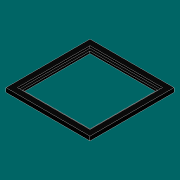
# Autodesk Inventor part: mirrorBackFrame
Saved by Autodesk Inventor 2016 (Build 200138000, 138)
## iProperties
Created: 2015-12-22
Part Number: mirrorBackFrame
Material: ABS Plastic
Document SubType Name: Modeling
Designer: sawai
Density: 1.06 g/cm^3
Appearance: Smooth - Black
Author: sawai
Autodesk Inventor part; units mm, degrees
ref_plane "YZ Plane" through (0, 0, 0) normal (1, 0, 0) x (0, 1, 0)
ref_plane "XZ Plane" through (0, 0, 0) normal (0, 1, 0) x (-1, 0, 0)
ref_plane "XY Plane" through (0, 0, 0) normal (0, 0, 1) x (1, 0, 0)
sketch "Sketch1" plane through (0, 0, 0) normal (0, 0, 1) x (1, 0, 0)
  line L0 (-57.15, 57.15) -> (57.15, 57.15) projected
  line L1 (57.15, 57.15) -> (57.15, -57.15) projected
  line L2 (57.15, -57.15) -> (-57.15, -57.15) projected
  line L3 (-57.15, -57.15) -> (-57.15, 57.15) projected
  line L4 (-63.5, -63.5) -> (63.5, -63.5) projected
  line L5 (63.5, -63.5) -> (63.5, 63.5) projected
  line L6 (63.5, 63.5) -> (-63.5, 63.5) projected
  line L7 (-63.5, 63.5) -> (-63.5, -63.5) projected
  point P0 (0, 0)
extrude "Extrusion1" add sketch "Sketch1" along normal blind 6.35 contours L0 L1 L2 L3 | L7 L6 L5 L4
sketch "Sketch2" plane through (0, 0, 6.35) normal (0, 0, 1) x (1, 0, 0)
  line L0 (50.9, 50.9) -> (-50.9, 50.9) projected
  line L1 (50.9, -50.9) -> (50.9, 50.9) projected
  line L2 (-50.9, -50.9) -> (50.9, -50.9) projected
  line L3 (-50.9, 50.9) -> (-50.9, -50.9) projected
  line L4 (-54.8688, 54.8688) -> (54.8688, 54.8688)
  line L5 (54.8688, 54.8688) -> (54.8688, -54.8688)
  line L6 (54.8688, -54.8688) -> (-54.8688, -54.8688)
  line L7 (-54.8688, -54.8688) -> (-54.8688, 54.8688)
  point P0 (0, 0)
  dimension "d2" = 3.9688
  constraints: 8 end point, 3 other
  measures "d2" distance between parallel lines of L0 L4
extrude "Extrusion2" cut sketch "Sketch2" against normal blind 3.175 contours L1 L2 L3 L0 | L4 L5 L6 L7
sketch "Sketch3" plane through (0, 0, 3.175) normal (0, 0, 1) x (1, 0, 0)
  line L0 (50.9, 50.9) -> (-50.9, 50.9) projected
  line L1 (-50.9, 50.9) -> (-50.9, -50.9) projected
  line L2 (50.9, -50.9) -> (50.9, 50.9) projected
  line L3 (-50.9, -50.9) -> (50.9, -50.9) projected
  point P0 (0, 0)
extrude "Extrusion3" cut sketch "Sketch3" against normal through all
equation "\"d0\" = plasticThickness"
equation "\"d2\" = 1.25 * mirrorThickness"
equation "\"d3\" = 0.5 * plasticThickness"
equation "\"d5\" = 0.5 * internalAcrylicThickness"
equation "\"frameAcrylicThickness\" = 9.525"
equation "\"internalAcrylicThickness\" = 6.35"
equation "\"height\" = 127"
equation "\"width\" = 127"
equation "\"depth\" = 120.142"
equation "\"mirrorAngle\" = 5deg"
equation "\"detectorWidth\" = 52"
equation "\"detectorHeight\" = 52"
equation "\"mirrorThickness\" = 3.175"
equation "\"fresnelThickness\" = 0.1"
equation "\"focalLength\" = 76.2"
equation "\"ior\" = 1.49"
equation "\"centerThickness\" = 1.524"
equation "\"fresnelAngle\" = 90deg"
equation "\"fresnelEffectiveDiameter\" = 152.4"
equation "\"oRingWidth\" = 1.5875"
equation "\"sensorHolderDepth\" = 19.05"
equation "\"aerogelClearence\" = 3.175"
equation "\"backplanePCBWidth\" = 76.2"
equation "\"backplanePCBHeight\" = 76.2"
equation "\"backplaneHoleOffsett\" = 6.35"
equation "\"backplanePostionOffsett\" = 12.7"
equation "\"moduleSlotClearence\" = 0.79375"
equation "\"plasticThickness\" = 6.35"
equation "\"aerogelHolderDepth\" = 37.30625"
equation "\"caseThickness\" = 6.35"
body "Solid1"
